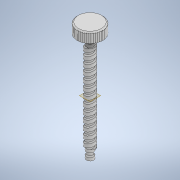
# Autodesk Inventor part: lead_screw
Saved by Autodesk Inventor 2021 (Build 250183000, 183)
## iProperties
Created: 2020-07-09
Part Number: lead_screw
Material: Generic
Document SubType Name: Modeling
Designer: Daniel
Density: 1 g/cm^3
Appearance: Default
Author: Daniel
Autodesk Inventor part; units mm, degrees
ref_plane "YZ Plane" through (0, 0, 0) normal (1, 0, 0) x (0, 1, 0)
ref_plane "XZ Plane" through (0, 0, 0) normal (0, 1, 0) x (-1, 0, 0)
ref_plane "XY Plane" through (0, 0, 0) normal (0, 0, 1) x (1, 0, 0)
sketch "Sketch1" plane through (0, 0, 0) normal (0, 1, 0) x (-1, 0, 0)
  circle A0 centre (0, 0) radius 4.95
  dimension "d0" = 9.9
  constraints: 1 centre point, 1 coincident
  measures "d0" diameter of A0
extrude "Extrusion1" add sketch "Sketch1" along normal blind 90
sketch "Sketch2" plane through (0, 0, 0) normal (0, 0, 1) x (-1, 0, 0)
  line L0 (4.95, 0) -> (4.95, 1.5)
  line L1 (4.95, 1.5) -> (3.651, 0.75) construction
  line L2 (4.95, 0) -> (3.651, 0.75)
  line L3 (-4.95, 0) -> (4.95, 0) construction
  line L4 (4.95, 0) -> (4.95, -90) projected
  line L5 (-4.95, -90) -> (-4.95, 0) projected
  line L6 (4.95, -90) -> (-4.95, -90) projected
  line L7 (4.95, 3.5) -> (3.651, 2.75)
  line L8 (3.651, 2.75) -> (3.651, 0.75)
  line L9 (4.95, 3.5) -> (4.95, 1.5)
  line L10 (-4.95, 0) -> (4.95, 0) projected
  point P0 (0, 0)
  dimension "d3" = 1.5
  dimension "d4" = 60
  dimension "d19" = 0
  dimension "d65" = 2
  constraints: 12 end point, 2 vertical, 1 collinear, 1 equal length, 1 parallel, 1 point on line
  measures "d3" distance of L0.start L0.end
  measures "d4" angle of L2 L1
  measures "d19" distance between parallel lines of L4 L0
  measures "d65" distance of L7.start L0.end
coil "Coil1" sketch "Sketch2" operation cut axis through (0, -10, 0) along (0, 1, 0) pitch 7 turns 13.857143 hand right contours L2 L8 L7 L9 L0
ref_plane "Work Plane1" through (0, 45, 0) normal (0, 1, 0) x (1, 0, 0)
sketch "Sketch8" plane through (0, 0, 0) normal (1, 0, 0) x (0, 1, 0)
  line L0 (90, 0) -> (100, 0)
  line L1 (100, 0) -> (100, -3.65)
  line L2 (100, -3.65) -> (90, -3.65)
  line L3 (90, -3.65) -> (90, 0)
  line L4 (92.9, -3.65) -> (97.1, -3.65)
  line L5 (97.1, -3.65) -> (97.1, -2.65)
  line L6 (97.1, -2.65) -> (92.9, -2.65)
  line L7 (92.9, -2.65) -> (92.9, -3.65)
  line L8 (90, -0.8124) -> (90, -0.8124) projected
  point P0 (0, 0)
  dimension "d50" = 10
  dimension "d51" = 3.65
  dimension "d52" = 4.2
  dimension "d53" = 2.9
  dimension "d54" = 1
  constraints: 16 end point, 4 parallel, 2 horizontal, 2 perpendicular, 2 point on line, 1 collinear
  measures "d50" distance of L1.end L2.end
  measures "d51" distance of L0.end L1.end
  measures "d52" distance of L5.end L6.end
  measures "d53" distance between parallel lines of L3 L7
  measures "d54" distance of L4.end L5.end
revolve "Revolution2" add sketch "Sketch8" angle 360 about axis through (0, 90, 0) along (0, 1, 0) contours L0 L1 L2 L5 L6 L7 L3
mirror "Mirror1" about plane through (0, 45, 0) normal (0, 1, 0) of "Revolution2"
sketch "Sketch7" plane through (0, 100, 0) normal (0, 1, 0) x (1, 0, 0)
  circle A0 centre (0, 0) radius 12.5
  circle A1 centre (0.2538, -11.9973) radius 1
  circle A2 centre (1.7555, -11.8709) radius 1
  circle A3 centre (3.2295, -11.5573) radius 1
  circle A4 centre (4.6525, -11.0614) radius 1
  circle A5 centre (6.0022, -10.391) radius 1
  circle A6 centre (7.2572, -9.5568) radius 1
  circle A7 centre (8.3978, -8.5719) radius 1
  circle A8 centre (9.4059, -7.4518) radius 1
  circle A9 centre (10.2657, -6.2142) radius 1
  circle A10 centre (10.9636, -4.8785) radius 1
  circle A11 centre (11.4886, -3.4659) radius 1
  circle A12 centre (11.8324, -1.9987) radius 1
  circle A13 centre (11.9896, -0.5) radius 1
  circle A14 centre (11.9577, 1.0067) radius 1
  circle A15 centre (11.7372, 2.4974) radius 1
  circle A16 centre (11.3317, 3.9488) radius 1
  circle A17 centre (10.7474, 5.3379) radius 1
  circle A18 centre (9.9936, 6.6428) radius 1
  circle A19 centre (9.0823, 7.843) radius 1
  circle A20 centre (8.0277, 8.9194) radius 1
  circle A21 centre (6.8465, 9.8552) radius 1
  circle A22 centre (5.5573, 10.6356) radius 1
  circle A23 centre (4.1805, 11.2483) radius 1
  circle A24 centre (2.7377, 11.6835) radius 1
  circle A25 centre (1.2518, 11.9345) radius 1
  circle A26 centre (-0.2538, 11.9973) radius 1
  circle A27 centre (-1.7555, 11.8709) radius 1
  circle A28 centre (-3.2295, 11.5573) radius 1
  circle A29 centre (-4.6525, 11.0614) radius 1
  circle A30 centre (-6.0022, 10.391) radius 1
  circle A31 centre (-7.2572, 9.5568) radius 1
  circle A32 centre (-8.3978, 8.5719) radius 1
  circle A33 centre (-9.4059, 7.4518) radius 1
  circle A34 centre (-10.2657, 6.2142) radius 1
  circle A35 centre (-10.9636, 4.8785) radius 1
  circle A36 centre (-11.4886, 3.4659) radius 1
  circle A37 centre (-11.8324, 1.9987) radius 1
  circle A38 centre (-11.9896, 0.5) radius 1
  circle A39 centre (-11.9577, -1.0067) radius 1
  circle A40 centre (-11.7372, -2.4974) radius 1
  circle A41 centre (-11.3317, -3.9488) radius 1
  circle A42 centre (-10.7474, -5.3379) radius 1
  circle A43 centre (-9.9936, -6.6428) radius 1
  circle A44 centre (-9.0823, -7.843) radius 1
  circle A45 centre (-8.0277, -8.9194) radius 1
  circle A46 centre (-6.8465, -9.8552) radius 1
  circle A47 centre (-5.5573, -10.6356) radius 1
  circle A48 centre (-4.1805, -11.2483) radius 1
  circle A49 centre (-2.7377, -11.6835) radius 1
  circle A50 centre (-1.2518, -11.9345) radius 1
  circle A51 centre (0, 0) radius 3.65 projected
  point P0 (1.0598, -12.5893)
  point P1 (2.6293, -12.3571)
  point P2 (4.1574, -11.9302)
  point P3 (5.6198, -11.315)
  point P4 (6.9937, -10.5215)
  point P5 (7.3978, -8.5668)
  point P6 (9.3905, -8.4517)
  point P7 (10.3757, -7.2081)
  point P8 (11.1973, -5.8508)
  point P9 (11.8424, -4.4013)
  point P10 (12.3006, -2.8823)
  point P11 (12.5649, -1.3179)
  point P12 (12.631, 0.2673)
  point P13 (12.4979, 1.8482)
  point P14 (12.1677, 3.4001)
  point P15 (11.6456, 4.8983)
  point P16 (10.9398, 6.3192)
  point P17 (10.0616, 7.6405)
  point P18 (9.0246, 8.8413)
  point P19 (7.8454, 9.9027)
  point P20 (6.5424, 10.8079)
  point P21 (5.1362, 11.5426)
  point P22 (3.649, 12.0953)
  point P23 (2.1043, 12.4573)
  point P24 (0.5264, 12.6228)
  point P25 (-1.0598, 12.5893)
  point P26 (-2.6293, 12.3571)
  point P27 (-4.1574, 11.9302)
  point P28 (-5.6198, 11.315)
  point P29 (-6.9937, 10.5215)
  point P30 (-8.2572, 9.562)
  point P31 (-9.3905, 8.4517)
  point P32 (-10.3757, 7.2081)
  point P33 (-11.1973, 5.8508)
  point P34 (-11.8424, 4.4013)
  point P35 (-12.3006, 2.8823)
  point P36 (-12.5649, 1.3179)
  point P37 (-12.631, -0.2673)
  point P38 (-12.4979, -1.8482)
  point P39 (-12.1677, -3.4001)
  point P40 (-11.6456, -4.8983)
  point P41 (-10.9398, -6.3192)
  point P42 (-10.0616, -7.6405)
  point P43 (-9.0246, -8.8413)
  point P44 (-7.8454, -9.9027)
  point P45 (-6.5424, -10.8079)
  point P46 (-5.1362, -11.5426)
  point P47 (-3.649, -12.0953)
  point P48 (-2.1043, -12.4573)
  point P49 (-0.5264, -12.6228)
  point P50 (-1.8853, -11.1607)
  point P51 (-0.4716, -11.309)
  point P52 (0.9495, -11.279)
  point P53 (2.3557, -11.071)
  point P54 (3.7247, -10.6885)
  point P55 (5.0349, -10.1374)
  point P56 (6.2658, -9.4264)
  point P57 (8.4132, -7.572)
  point P58 (9.2958, -6.4579)
  point P59 (10.0319, -5.2419)
  point P60 (10.6098, -3.9432)
  point P61 (11.0203, -2.5823)
  point P62 (11.2571, -1.1808)
  point P63 (11.3163, 0.2394)
  point P64 (11.1971, 1.6559)
  point P65 (10.9013, 3.0462)
  point P66 (10.4335, 4.3884)
  point P67 (9.8012, 5.6615)
  point P68 (9.0144, 6.8453)
  point P69 (8.0853, 7.9211)
  point P70 (7.0288, 8.872)
  point P71 (5.8614, 9.683)
  point P72 (4.6016, 10.3413)
  point P73 (3.2692, 10.8365)
  point P74 (1.8853, 11.1607)
  point P75 (0.4716, 11.309)
  point P76 (-0.9495, 11.279)
  point P77 (-2.3557, 11.071)
  point P78 (-3.7247, 10.6885)
  point P79 (-5.0349, 10.1374)
  point P80 (-6.2658, 9.4264)
  point P81 (-7.3978, 8.5668)
  point P82 (-8.4132, 7.572)
  point P83 (-9.2958, 6.4579)
  point P84 (-10.0319, 5.2419)
  point P85 (-10.6098, 3.9432)
  point P86 (-11.0203, 2.5823)
  point P87 (-11.2571, 1.1808)
  point P88 (-11.3163, -0.2394)
  point P89 (-11.1971, -1.6559)
  point P90 (-10.9013, -3.0462)
  point P91 (-10.4335, -4.3884)
  point P92 (-9.8012, -5.6615)
  point P93 (-9.0144, -6.8453)
  point P94 (-8.0853, -7.9211)
  point P95 (-7.0288, -8.872)
  point P96 (-5.8614, -9.683)
  point P97 (-4.6016, -10.3413)
  point P98 (-3.2692, -10.8365)
  point P99 (8.2572, -9.562)
  dimension "d39" = 2
  dimension "d40" = 25
  dimension "d41" = 12
  dimension "d44" = 360
  constraints: 51 centre point, 2 coincident, 101 other
  measures "d39" diameter of A1
  measures "d40" diameter of A0
  measures "d41" distance of A0.centre A1.centre
extrude "Extrusion5" add sketch "Sketch7" along normal blind 10 contours A0 A12 A13 A14 | A0 A14 A13 A12 | A14 A13 A0 | A0 A13 A14 | A12 A13 A0 | A0 A13 A12 | A13 A14 A15 A0 | A0 A15 A14 A13 | A13 A12 A11 A10 A9 A8 A7 A6 A5 A4 A3 A2 A1 A50 A49 A48 A47 A46 A45 A44 A43 A42 A41 A40 A39 A38 A37 A36 A35 A34 A33 A32 A31 A30 A29 A28 A27 A26 A25 A24 A23 A22 A21 A20 A19 A18 A17 A16 A15 A14 | A13 A12 A11 A0 | A0 A11 A12 A13 | A15 A14 A0 | A0 A14 A15 | A15 A16 A0 A14 | A11 A12 A0 | A0 A12 A11 | A12 A0 A10 A11 | A0 A16 A15 A14 | A16 A17 A0 A15 | A15 A0 A16 | A12 A11 A10 A0 | A11 A0 A9 A10 | A10 A0 A11 | A0 A15 A16 | A0 A17 A16 A15 | A17 A18 A0 A16 | A16 A0 A17 | A10 A11 A0 | A10 A0 A8 A9 | A9 A0 A10 | A11 A10 A9 A0 | A0 A16 A17 | A0 A18 A17 A16 | A18 A19 A0 A17 | A17 A0 A18 | A9 A10 A0 | A9 A0 A7 A8 | A8 A0 A9 | A10 A9 A8 A0 | A0 A17 A18 | A0 A19 A18 A17 | A19 A20 A0 A18 | A18 A0 A19 | A8 A9 A0 | A8 A0 A6 A7 | A7 A0 A8 | A9 A8 A7 A0 | A0 A18 A19 | A0 A20 A19 A18 | A20 A21 A0 A19 | A19 A0 A20 | A7 A8 A0 | A7 A0 A5 A6 | A6 A0 A7 | A8 A7 A6 A0 | A0 A19 A20 | A0 A21 A20 A19 | A21 A22 A0 A20 | A20 A0 A21 | A6 A7 A0 | A6 A0 A4 A5 | A5 A0 A6 | A7 A6 A5 A0 | A0 A20 A21 | A0 A22 A21 A20 | A22 A23 A0 A21 | A21 A0 A22 | A5 A6 A0 | A5 A0 A3 A4 | A4 A0 A5 | A6 A5 A4 A0 | A0 A21 A22 | A0 A23 A22 A21 | A23 A24 A0 A22 | A22 A0 A23 | A4 A0 A2 A3 | A3 A0 A4 | A5 A4 A3 A0 | A0 A4 A5 | A0 A22 A23 | A0 A24 A23 A22 | A24 A25 A0 A23 | A23 A0 A24 | A3 A0 A1 A2 | A2 A0 A3 | A4 A3 A2 A0 | A0 A3 A4 | A0 A23 A24 | A0 A25 A24 A23 | A25 A26 A0 A24 | A24 A0 A25 | A2 A0 A50 A1 | A1 A0 A2 | A3 A2 A1 A0 | A0 A2 A3 | A0 A24 A25 | A0 A26 A25 A24 | A26 A27 A0 A25 | A25 A0 A26 | A50 A0 A1 | A1 A0 A49 A50 | A2 A1 A50 A0 | A0 A1 A2 | A0 A25 A26 | A0 A27 A26 A25 | A27 A28 A0 A26 | A26 A0 A27 | A1 A50 A49 A0 | A0 A50 A1 | A50 A0 A48 A49 | A49 A0 A50 | A0 A26 A27 | A0 A28 A27 A26 | A28 A29 A0 A27 | A27 A0 A28 | A49 A50 A0 | A49 A0 A47 A48 | A48 A0 A49 | A50 A49 A48 A0 | A0 A27 A28 | A0 A29 A28 A27 | A29 A30 A0 A28 | A28 A0 A29 | A48 A0 A46 A47 | A47 A0 A48 | A49 A48 A47 A0 | A0 A48 A49 | A0 A28 A29 | A0 A30 A29 A28 | A30 A31 A0 A29 | A29 A0 A30 | A47 A0 A45 A46 | A46 A0 A47 | A48 A47 A46 A0 | A0 A47 A48 | A0 A29 A30 | A0 A31 A30 A29 | A31 A32 A0 A30 | A30 A0 A31 | A46 A0 A44 A45 | A45 A0 A46 | A47 A46 A45 A0 | A0 A46 A47 | A0 A30 A31 | A0 A32 A31 A30 | A32 A33 A0 A31 | A31 A0 A32 | A45 A0 A43 A44 | A44 A0 A45 | A46 A45 A44 A0 | A0 A45 A46 | A0 A31 A32 | A0 A33 A32 A31 | A33 A34 A0 A32 | A32 A0 A33 | A44 A45 A0 | A45 A44 A43 A0 | A0 A32 A33 | A0 A34 A33 A32 | A44 A0 A42 A43 | A43 A0 A44 | A43 A44 A0 | A34 A33 A0 | A0 A33 A34 | A34 A35 A0 A33 | A43 A42 A0 A44 | A33 A0 A35 A34 | A43 A0 A42 | A42 A41 A0 A43 | A43 A0 A41 A42 | A42 A0 A43 | A35 A0 A34 | A34 A0 A36 A35 | A35 A34 A0 | A35 A36 A0 A34 | A42 A0 A41 | A41 A40 A0 A42 | A36 A0 A35 | A35 A0 A37 A36 | A41 A0 A40 | A40 A39 A0 A41 | A0 A42 A41 | A0 A40 A41 A42 | A36 A35 A0 | A35 A36 A37 A0 | A37 A0 A36 | A36 A0 A38 A37 | A40 A0 A39 | A39 A38 A0 A40 | A0 A41 A40 | A0 A39 A40 A41 | A37 A36 A0 | A36 A37 A38 A0 | A38 A0 A37 | A37 A0 A39 A38 | A39 A0 A38 | A0 A40 A39 | A0 A38 A39 A40 | A38 A37 A0 | A37 A38 A39 A0 | A0 A39 A38 | A51
fillet "Fillet1" radius 2 1 edges at (0, 100, 3.65)
chamfer "Chamfer4" distance 1 angle 45 2 edges at (0, 92.9, 2.65) (0, -7.1, 2.65)
sketch "Sketch9" plane through (0, 0, 0) normal (1, 0, 0) x (0, 1, 0)
  line L0 (108, 13.65) -> (112.2325, 9.4175)
  line L1 (108, 13.65) -> (113.9857, 13.65) construction
  line L2 (112.2325, 9.4175) -> (112.2325, 13.65)
  line L3 (100, 12.3571) -> (110, 12.3571) projected
  line L4 (112.2325, 13.65) -> (108, 13.65)
  line L5 (97.1, 3.65) -> (97.1, -3.65) projected
  line L6 (97.1, 0) -> (124.7436, 0)
  line L7 (98, -3.65) -> (98, 3.65) projected
  point P0 (0, 0)
  dimension "d63" = 45
  dimension "d66" = 10
  dimension "d67" = 10
  constraints: 10 end point, 2 horizontal, 2 perpendicular, 1 equal length, 1 midpoint
  measures "d63" angle of L0 L1
  measures "d66" distance from line of L7 L0.start
  measures "d67" horizontal distance of L7.end L0.start
revolve "Revolution3" cut sketch "Sketch9" angle 360 about axis through (0, 97.1, 0) along (0, 1, 0)
equation "\"d1\" = length"
equation "\"d8\" = pitch"
equation "\"d9\" = pitch + length"
equation "\"pitch\" = 7"
equation "\"length\" = 90"
body "Solid1"
